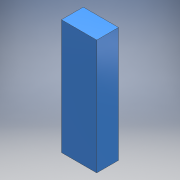
# Autodesk Inventor part: bateria
Saved by Autodesk Inventor 2017 (Build 210142000, 142)
## iProperties
Part Number: bateria
Material: Genérico
Document SubType Name: Modeling
Designer: Roberto
Density: 1 g/cm^3
Appearance: Valor por defecto
Author: Roberto
Autodesk Inventor part; units mm, degrees
ref_plane "YZ Plane" through (0, 0, 0) normal (1, 0, 0) x (0, 1, 0)
ref_plane "XZ Plane" through (0, 0, 0) normal (0, 1, 0) x (-1, 0, 0)
ref_plane "XY Plane" through (0, 0, 0) normal (0, 0, 1) x (1, 0, 0)
sketch "Boceto1" plane through (0, 0, 0) normal (0, 1, 0) x (-1, 0, 0)
  line L0 (0, 0) -> (4.2, 0)
  line L1 (4.2, 0) -> (4.2, -13.7)
  line L2 (4.2, -13.7) -> (0, -13.7)
  line L3 (0, -13.7) -> (0, 0)
  constraints: 8 end point
extrude "Extrusión1" add sketch "Boceto1" along normal blind 2.6
